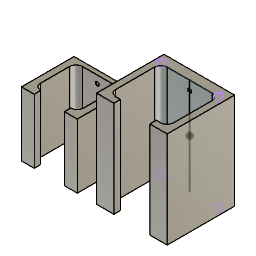
Drill Mounts (Autodesk Fusion 360 design; units mm, degrees)
Autodesk Fusion 360 part; units mm, degrees
sketch "Sketch1" plane through (0, 0, 0) normal (0, 0, 1) x (1, 0, 0)
  line L0 (0, 0) -> (90, 0)
  line L1 (90, 0) -> (90, 80)
  line L2 (90, 80) -> (0, 80)
  line L3 (0, 80) -> (0, 0)
  line L4 (0, 0) -> (17, 0)
  line L5 (17, 0) -> (17, -10)
  line L6 (17, -10) -> (0, -10)
  line L7 (0, -10) -> (0, 0)
  line L8 (90, 0) -> (73, 0)
  line L9 (73, 0) -> (73, -10)
  line L10 (73, -10) -> (90, -10)
  line L11 (90, -10) -> (90, 0)
  line L12 (0, -10) -> (-10, -10)
  line L13 (-10, -10) -> (-10, 80)
  line L14 (-10, 80) -> (0, 80)
  line L15 (0, 80) -> (0, -10)
  line L16 (85, -10) -> (90, -10)
  line L17 (90, -10) -> (90, 80)
  line L18 (90, -10) -> (100, -10)
  line L19 (100, -10) -> (100, 80)
  line L20 (100, 80) -> (90, 80)
  line L21 (90, 80) -> (90, -10)
  line L22 (-10, 80) -> (100, 80)
  line L23 (100, 80) -> (100, 95)
  line L24 (100, 95) -> (-10, 95)
  line L25 (-10, 95) -> (-10, 80)
  dimension "d1" = 90
  dimension "d2" = 80
  dimension "d3" = 17
  dimension "d4" = 10
  dimension "d5" = 17
  dimension "d6" = 10
  dimension "d7" = 10
  dimension "d8" = 90
  constraint horizontal L0
  constraint vertical L1
  constraint horizontal L2
  constraint vertical L3
  constraint coincident L0.start L3.end
  constraint horizontal L4
  constraint vertical L5
  constraint horizontal L6
  constraint vertical L7
  constraint horizontal L8
  constraint vertical L9
  constraint horizontal L10
  constraint vertical L11
  constraint horizontal L12
  constraint vertical L13
  constraint horizontal L14
  constraint vertical L15
  constraint horizontal L16
  constraint vertical L17
  constraint horizontal L18
  constraint vertical L19
  constraint horizontal L20
  constraint vertical L21
  constraint horizontal L22
  constraint vertical L23
  constraint horizontal L24
  constraint vertical L25
  measures "d1" distance of L0.start L0.end
  measures "d2" distance of L0.start L2.end
  measures "d3" distance of L0.start L4.end
  measures "d4" distance of L0.start L6.end
  measures "d5" distance of L0.end L8.end
  measures "d6" distance of L0.end L10.end
  measures "d7" distance of L6.end L12.end
  measures "d8" distance of L6.end L2.end
extrude "Extrude1" add sketch "Sketch1" along normal blind 150 contours L3 L7 L12 L13 L14 L15 L22 | L0 L4 L5 L6 L7 L15 | L2 L14 L20 L22 L23 L24 L25 | L0 L8 L9 L10 L11 L16 L17 L21 | L1 L11 L17 L18 L19 L20 L21 L22 makes body 1
hole "Hole1" at (45, 80, 75) direction (0, 1, 0) diameter 4.2 depth 20 tip angle 118 countersink diameter 6 countersink angle 90 bodies 1
sketch "Sketch2" plane through (0, 80, 0) normal (0, -1, 0) x (1, 0, 0)
  circle A0 centre (45, 75) radius 3
  line L0 (0, 0) -> (90, 0)
  line L1 (90, 0) -> (90, 150)
  line L2 (90, 150) -> (0, 150)
  line L3 (0, 150) -> (0, 0)
  line L4 (45, 75) -> (45, 150)
  line L5 (45, 75) -> (45, 0)
  constraint coincident A0.centre L4.start
  constraint midpoint L2 L4.end
  constraint midpoint L0 L5.end
hole "Hole2" at (45.0217, 80, 135.9855) direction (0, 1, 0) diameter 4.2 depth 20 tip angle 118 countersink diameter 6 countersink angle 90 bodies 1
hole "Hole3" at (44.9841, 80, 10.2643) direction (0, 1, 0) diameter 4.2 depth 20 tip angle 118 countersink diameter 6 countersink angle 90 bodies 1
sketch "Sketch3" plane through (0, 0, 0) normal (0, 0, 1) x (1, 0, 0)
  line L0 (-50, 0) -> (-117, 0)
  line L1 (-117, 0) -> (-117, 65)
  line L2 (-117, 65) -> (-50, 65)
  line L3 (-50, 65) -> (-50, 0)
  line L4 (-117, 0) -> (-107, 0)
  line L5 (-107, 0) -> (-107, -10)
  line L6 (-107, -10) -> (-117, -10)
  line L7 (-117, -10) -> (-117, 0)
  line L8 (-50, 0) -> (-60, 0)
  line L9 (-60, 0) -> (-60, -10)
  line L10 (-60, -10) -> (-50, -10)
  line L11 (-50, -10) -> (-50, 0)
  line L12 (-117, 65) -> (-127, 65)
  line L13 (-127, 65) -> (-127, -10)
  line L14 (-127, -10) -> (-117, -10)
  line L15 (-117, -10) -> (-117, 65)
  line L16 (-50, 65) -> (-40, 65)
  line L17 (-40, 65) -> (-40, -10)
  line L18 (-40, -10) -> (-50, -10)
  line L19 (-50, -10) -> (-50, 65)
  line L20 (-127, 65) -> (-40, 65)
  line L21 (-40, 65) -> (-40, 72)
  line L22 (-40, 72) -> (-127, 72)
  line L23 (-127, 72) -> (-127, 65)
  dimension "d27" = 67
  dimension "d28" = 65
  dimension "d29" = 10
  dimension "d30" = 10
  dimension "d31" = 10
  dimension "d32" = 7
  constraint horizontal L0
  constraint vertical L1
  constraint horizontal L2
  constraint vertical L3
  constraint horizontal L4
  constraint vertical L5
  constraint horizontal L6
  constraint vertical L7
  constraint horizontal L8
  constraint vertical L9
  constraint horizontal L10
  constraint vertical L11
  constraint horizontal L12
  constraint vertical L13
  constraint horizontal L14
  constraint vertical L15
  constraint horizontal L16
  constraint vertical L17
  constraint horizontal L18
  constraint vertical L19
  constraint horizontal L20
  constraint vertical L21
  constraint horizontal L22
  constraint vertical L23
  measures "d27" distance of L0.start L0.end
  measures "d28" distance of L0.start L2.end
  measures "d29" distance of L0.end L4.end
  measures "d30" distance of L0.end L6.end
  measures "d31" distance of L1.end L12.end
  measures "d32" distance of L12.end L22.end
extrude "Extrude2" add sketch "Sketch3" along normal blind 100 separate body contours L0 L8 L9 L10 L11 L19 | L3 L11 L16 L17 L18 L19 L20 | L2 L12 L16 L20 L21 L22 L23 | L0 L4 L5 L6 L7 L15 | L1 L7 L12 L13 L14 L15 L20 makes body 2
fillet "Fillet1" radius 10 8 edges at (0, 80, 75) (0, 0, 75) (90, 0, 75) (90, 80, 75) (-117, 65, 50) (-50, 65, 50) (-117, 0, 50) (-50, 0, 50) on bodies 1 2
hole "Hole4" at (-83.9041, 65, 88.2242) direction (0, 1, 0) diameter 4.2 depth 10 tip angle 118 countersink diameter 6 countersink angle 90 bodies 2
hole "Hole5" at (-83.6647, 65, 14.2796) direction (0, 1, 0) diameter 4.2 depth 10 tip angle 118 countersink diameter 6 countersink angle 90 bodies 2
